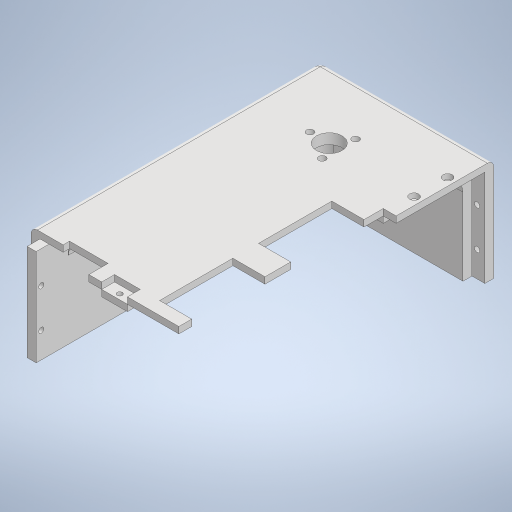
# Autodesk Inventor part: top_2
Saved by Autodesk Inventor 2023 (Build 270158000, 158)
## iProperties
Created: 2024-04-26
Part Number: top_2
Material: 常规
Document SubType Name: Modeling
Designer: Nitrene.P.L
Density: 1 g/cm^3
Appearance: 默认
Author: Nitrene.P.L
Autodesk Inventor part; units mm, degrees
ref_plane "YZ Plane" through (0, 0, 0) normal (1, 0, 0) x (0, 1, 0)
ref_plane "XZ Plane" through (0, 0, 0) normal (0, 1, 0) x (-1, 0, 0)
ref_plane "XY Plane" through (0, 0, 0) normal (0, 0, 1) x (1, 0, 0)
sketch "草图6" plane through (0, 0, 0) normal (0, 1, 0) x (-1, 0, 0)
  line L0 (125, 235) -> (-125, 235)
  line L1 (-125, 235) -> (-125, -235)
  line L2 (-125, -235) -> (125, -235)
  line L3 (125, -235) -> (125, 235)
  line L4 (0, 3) -> (0, -5)
  line L5 (3.5058, 0) -> (-3.4421, 0)
  line L6 (25, 144) -> (-32, 144)
  line L7 (-32, 144) -> (-32, 87)
  line L8 (-32, 87) -> (25, 87)
  line L9 (25, 87) -> (25, 144)
  line L10 (25, 67) -> (-32, 67)
  line L11 (-32, 67) -> (-32, 10)
  line L12 (-32, 10) -> (25, 10)
  line L13 (25, 10) -> (25, 67)
  line L14 (25, -10) -> (-32, -10)
  line L15 (-32, -10) -> (-32, -67)
  line L16 (-32, -67) -> (25, -67)
  line L17 (25, -67) -> (25, -10)
  line L18 (25, -87) -> (-32, -87)
  line L19 (-32, -87) -> (-32, -144)
  line L20 (-32, -144) -> (25, -144)
  line L21 (25, -144) -> (25, -87)
  line L22 (-66, 100) -> (-95, 100)
  line L23 (-95, 100) -> (-95, 54)
  line L24 (-95, 54) -> (-66, 54)
  line L25 (-66, 54) -> (-66, 100)
  line L26 (-66, -54) -> (-95, -54)
  line L27 (-95, -54) -> (-95, -100)
  line L28 (-95, -100) -> (-66, -100)
  line L29 (-66, -100) -> (-66, -54)
  line L30 (100, 15) -> (70, 15)
  line L31 (70, 15) -> (70, -15)
  line L32 (70, -15) -> (100, -15)
  line L33 (100, -15) -> (100, 15)
  circle A0 centre (65, 182) radius 10
  circle A1 centre (65, -182) radius 10
  circle A2 centre (65, 182) radius 15
  circle A3 centre (80, 182) radius 1.5
  circle A4 centre (57.5, 194.9904) radius 1.5
  circle A5 centre (57.5, 169.0096) radius 1.5
  line L34 (125, 235) -> (0, 235)
  line L35 (0, 235) -> (0, 0)
  line L36 (0, 0) -> (125, 0)
  line L37 (125, 0) -> (125, 235)
  line L38 (-125, 235) -> (0, 235)
  line L39 (0, 235) -> (0, 0)
  line L40 (0, 0) -> (-125, 0)
  line L41 (-125, 0) -> (-125, 235)
  line L42 (-125, -235) -> (0, -235)
  line L43 (0, -235) -> (0, 0)
  line L44 (0, 0) -> (-125, 0)
  line L45 (-125, 0) -> (-125, -235)
  line L46 (125, -235) -> (0, -235)
  line L47 (0, -235) -> (0, 0)
  line L48 (0, 0) -> (125, 0)
  line L49 (125, 0) -> (125, -235)
  circle A6 centre (65, -182) radius 15
  circle A7 centre (80, -182) radius 1.5
  circle A8 centre (57.5, -169.0096) radius 1.5
  circle A9 centre (57.5, -194.9904) radius 1.5
  point P0 (70, 0)
  point P1 (0, -10)
  point P2 (0, -67)
  point P3 (0, -87)
  point P4 (0, -144)
  point P5 (0, -235)
  point P6 (100, 0)
  dimension "d153" = 30
  dimension "d156" = 30
  dimension "d122" = 470
  dimension "d123" = 250
  dimension "d124" = 57
  dimension "d125" = 57
  dimension "d126" = 57
  dimension "d127" = 57
  dimension "d128" = 57
  dimension "d129" = 57
  dimension "d130" = 57
  dimension "d131" = 57
  dimension "d132" = 91
  dimension "d133" = 20
  dimension "d134" = 20
  dimension "d135" = 20
  dimension "d136" = 93
  dimension "d137" = 29
  dimension "d138" = 46
  dimension "d139" = 46
  dimension "d140" = 135
  dimension "d141" = 108
  dimension "d142" = 30
  dimension "d143" = 30
  dimension "d144" = 30
  dimension "d145" = 25
  dimension "d146" = 220
  dimension "d147" = 20
  dimension "d148" = 53
  dimension "d149" = 60
  dimension "d150" = 20
  dimension "d151" = 53
  dimension "d152" = 60
  dimension "d154" = 3
  dimension "d155" = 360
  dimension "d157" = 3
  dimension "d158" = 360
  constraints: 100 end point, 24 parallel, 14 horizontal, 12 perpendicular, 8 centre point, 3 collinear, 2 coincident, 2 horizontal alignment, 2 point on line, 2 vertical, 20 other
  measures "d122" distance of L3.start L3.end
  measures "d123" distance of L3.end L1.start
  measures "d124" distance of L8.end L8.start
  measures "d125" distance of L8.start L6.end
  measures "d126" distance of L13.start L11.end
  measures "d127" distance of L11.end L11.start
  measures "d128" distance of L16.end L15.end
  measures "d129" distance of L15.end L14.end
  measures "d130" distance of L20.end L19.end
  measures "d131" distance of L19.end L19.start
  measures "d132" distance between parallel lines of L0 L6
  measures "d133" distance between parallel lines of L10 L8
  measures "d134" distance between parallel lines of L12 L14
  measures "d135" distance between parallel lines of L18 L16
  measures "d136" distance between parallel lines of L1 L7
  measures "d137" distance of L25.start L23.end
  measures "d138" distance of L23.end L22.end
  measures "d139" distance of L27.end L27.start
  measures "d140" distance between parallel lines of L0 L22
  measures "d141" distance between parallel lines of L26 L24
  measures "d142" distance between parallel lines of L1 L23
  measures "d143" distance of L32.end L31.end
  measures "d144" distance of L31.end L31.start
  measures "d145" distance between parallel lines of L3 L33
  measures "d146" distance between parallel lines of L0 L30
  measures "d147" diameter of A0
  measures "d148" distance from line of L0 A0.centre
  measures "d149" distance from line of L3 A0.centre
  measures "d150" diameter of A1
  measures "d151" distance from line of L2 A1.centre
  measures "d152" distance from line of L3 A1.centre
  measures "d154" diameter of A3
  measures "d157" diameter of A7
extrude "拉伸5" add sketch "草图6" along normal blind 10 contours L3 L2 L43 L20 L21 L18 L16 L17 L14 L4 L5 L36 L31 L32 L33 | A7 A6 A9 A8
sketch "草图7" plane through (0, 0, 0) normal (0, -1, 0) x (1, 0, 0)
  line L0 (-70, 0) -> (0, 0) projected
  line L1 (0, 0) -> (-40, 0)
  line L2 (-40, 0) -> (-40, -159)
  line L3 (-40, -159) -> (0, -159)
  line L4 (0, -159) -> (0, 0)
  line L5 (-25, -144) -> (0, -144) projected
  line L6 (-25, -87) -> (-25, -144) projected
  line L7 (-60, 0) -> (-111, 0)
  line L8 (-111, 0) -> (-111, -25)
  line L9 (-111, -25) -> (-60, -25)
  line L10 (-60, -25) -> (-60, 0)
  line L11 (-70, -15) -> (-70, 0) projected
  line L12 (-100, -15) -> (-70, -15) projected
  line L13 (-100, 0) -> (-100, -15) projected
  dimension "d161" = 15
  dimension "d162" = 15
  dimension "d163" = 10
  dimension "d164" = 10
  dimension "d165" = 11
  constraints: 16 end point, 4 parallel, 2 horizontal, 2 perpendicular, 1 point on line
  measures "d161" distance between parallel lines of L5 L3
  measures "d162" distance between parallel lines of L6 L2
  measures "d163" distance between parallel lines of L10 L11
  measures "d164" distance between parallel lines of L9 L12
  measures "d165" distance between parallel lines of L13 L8
extrude "拉伸6" cut sketch "草图7" against normal blind 5 contours L0 L10 L9 L8 L7 L13 L12 L11 | L0 L4 L3 L2
sketch "草图8" plane through (0, 0, 0) normal (0, -1, 0) x (1, 0, 0)
  line L0 (-125, 0) -> (-111, 0) projected
  line L1 (-125, -235) -> (-125, 0) projected
  line L2 (-111, 0) -> (-125, 0)
  line L3 (-125, 0) -> (-125, -235)
  line L4 (-125, -235) -> (-111, -235)
  line L5 (-111, -235) -> (-111, 0)
  line L6 (0, -235) -> (-125, -235) projected
  line L7 (0, -235) -> (-125, -235)
  line L8 (-125, -235) -> (-125, -221)
  line L9 (-125, -221) -> (0, -221)
  line L10 (0, -221) -> (0, -235)
  point P0 (0, 0)
  point P1 (-111, -221)
  dimension "d168" = 14
  constraints: 16 end point, 4 parallel, 2 horizontal, 2 perpendicular, 1 point on line
  measures "d168" distance of L7.end L8.end
extrude "拉伸7" add sketch "草图8" along normal blind 70
sketch "草图11" plane through (0, 10, 0) normal (0, 1, 0) x (1, 0, 0)
  line L0 (-60, 0) -> (-60, 25) projected
  line L1 (-60, 0) -> (-40, 0)
  line L2 (-40, 0) -> (-40, 10)
  line L3 (-40, 10) -> (-60, 10)
  line L4 (-60, 10) -> (-60, 0)
  line L5 (-100, 0) -> (-100, 15) projected
  line L6 (-125, 235) -> (-125, 0) projected
  line L7 (-100, 0) -> (-125, 0)
  line L8 (-125, 0) -> (-125, 10)
  line L9 (-125, 10) -> (-100, 10)
  line L10 (-100, 10) -> (-100, 0)
  point P0 (0, 0)
  dimension "d178" = 10
  dimension "d179" = 20
  dimension "d187" = 10
  constraints: 16 end point, 4 parallel, 2 horizontal, 2 perpendicular, 1 point on line
  measures "d178" distance of L2.end L1.end
  measures "d179" distance between parallel lines of L0 L2
  measures "d187" distance of L7.end L8.end
extrude "拉伸9" cut sketch "草图11" against normal blind 5
sketch "草图12" plane through (0, 5, 0) normal (0, 1, 0) x (1, 0, 0)
  circle A0 centre (-50, 4) radius 2.1
  line L0 (-40, 0) -> (-60, 0) projected
  line L1 (-40, 10) -> (-40, 0) projected
  point P0 (0, 0)
  dimension "d182" = 4.2
  dimension "d183" = 4
  dimension "d184" = 10
  constraints: 1 centre point
  measures "d182" diameter of A0
  measures "d183" distance from line of L0 A0.centre
  measures "d184" distance from line of L1 A0.centre
extrude "拉伸10" cut sketch "草图12" against normal blind 5
sketch "草图13" plane through (-125, -70, -235) normal (-1, 0, 0) x (0, 0, 1)
  line L0 (235, 75) -> (225, 75) projected
  line L1 (235, 75) -> (225, 75)
  line L2 (225, 75) -> (225, 0)
  line L3 (225, 0) -> (235, 0)
  line L4 (235, 0) -> (235, 75)
  point P0 (235, 70)
  dimension "d188" = 10
  constraints: 8 end point, 2 parallel, 1 horizontal, 1 perpendicular
  measures "d188" distance between parallel lines of L2 L4
extrude "拉伸11" cut sketch "草图13" against normal blind 7
sketch "草图14" plane through (-118, -70, -235) normal (-1, 0, 0) x (0, 0, 1)
  circle A0 centre (231, 50) radius 2.1
  circle A1 centre (231, 20) radius 2.1
  line L0 (0, 80) -> (225, 80) projected
  line L1 (225, 0) -> (0, 0) projected
  line L2 (235, 75) -> (235, 0) projected
  point P0 (235, 70)
  dimension "d191" = 4.2
  dimension "d192" = 4.2
  dimension "d193" = 30
  dimension "d194" = 20
  dimension "d195" = 4
  dimension "d196" = 4
  constraints: 2 centre point
  measures "d191" diameter of A0
  measures "d192" diameter of A1
  measures "d193" distance from line of L0 A0.centre
  measures "d194" distance from line of L1 A1.centre
  measures "d195" distance from line of L2 A0.centre
  measures "d196" distance from line of L2 A1.centre
extrude "拉伸12" cut sketch "草图14" against normal blind 7
fillet "圆角1" radius 10 3 edges at (-111, 0, -123) (-111, -35, -221) (-55.5, 0, -221)
sketch "草图15" plane through (0, 10, 0) normal (0, 1, 0) x (1, 0, 0)
  line L0 (0, 159) -> (0, 211) projected
  line L1 (0, 159) -> (10, 159)
  line L2 (10, 159) -> (10, 235)
  line L3 (10, 235) -> (0, 235)
  line L4 (0, 235) -> (0, 159)
  circle A0 centre (4, 179) radius 2.1
  circle A1 centre (4, 205) radius 2.1
  point P0 (0, 0)
  point P1 (0, 211)
  dimension "d201" = 10
  dimension "d202" = 4.2
  dimension "d203" = 4.2
  dimension "d204" = 6
  dimension "d205" = 6
  dimension "d206" = 76
  dimension "d207" = 30
  dimension "d208" = 20
  constraints: 8 end point, 2 centre point, 2 parallel, 1 horizontal, 1 perpendicular
  measures "d201" distance of L3.end L2.end
  measures "d202" diameter of A0
  measures "d203" diameter of A1
  measures "d204" distance from line of L2 A0.centre
  measures "d205" distance from line of L2 A1.centre
  measures "d206" distance between parallel lines of L3 L1
  measures "d207" distance from line of L3 A1.centre
  measures "d208" distance from line of L1 A0.centre
extrude "拉伸13" add sketch "草图15" against normal blind 5
sketch "草图16" plane through (0, -70, -235) normal (0, 0, -1) x (-1, 0, 0)
  line L0 (-10, 75) -> (0, 75) projected
  line L1 (0, 60) -> (0, 0) projected
  line L2 (-10, 75) -> (0, 75)
  line L3 (0, 75) -> (0, 0)
  line L4 (0, 0) -> (-10, 0)
  line L5 (-10, 0) -> (-10, 75)
  circle A0 centre (-4, 50) radius 2.1
  circle A1 centre (-4, 20) radius 2.1
  line L6 (-10, 80) -> (125, 80) projected
  line L7 (125, 0) -> (0, 0) projected
  point P0 (0, 70)
  point P1 (0, 75)
  dimension "d211" = 4.2
  dimension "d212" = 4.2
  dimension "d213" = 30
  dimension "d214" = 20
  dimension "d215" = 6
  dimension "d216" = 6
  constraints: 8 end point, 2 centre point, 2 parallel, 1 horizontal, 1 perpendicular
  measures "d211" diameter of A0
  measures "d212" diameter of A1
  measures "d213" distance from line of L6 A0.centre
  measures "d214" distance from line of L7 A1.centre
  measures "d215" distance from line of L5 A0.centre
  measures "d216" distance from line of L5 A1.centre
extrude "拉伸14" add sketch "草图16" against normal blind 7
sketch "草图17" plane through (0, 10, 0) normal (0, 1, 0) x (1, 0, 0)
  circle A0 centre (4, 179) radius 2.1 projected
  circle A1 centre (4, 179) radius 3.6
  circle A2 centre (4, 205) radius 2.1 projected
  circle A3 centre (4, 205) radius 3.6
  point P0 (0, 0)
  dimension "d219" = 7.2
  dimension "d220" = 7.2
  constraints: 2 centre point, 2 coincident
  measures "d219" diameter of A1
  measures "d220" diameter of A3
extrude "拉伸15" cut sketch "草图17" against normal blind 4
sketch "草图18" plane through (-125, -70, -235) normal (0, 0, -1) x (-1, 0, 0)
  circle A0 centre (-129, 50) radius 2.1 projected
  circle A1 centre (-129, 50) radius 3.6
  circle A2 centre (-129, 20) radius 2.1 projected
  circle A3 centre (-129, 20) radius 3.6
  point P0 (-125, 70)
  dimension "d223" = 7.2
  dimension "d224" = 7.2
  constraints: 2 centre point, 2 coincident
  measures "d223" diameter of A1
  measures "d224" diameter of A3
extrude "拉伸16" cut sketch "草图18" against normal blind 4
fillet "圆角3" radius 5 3 edges at (-57.5, 10, -235) (-125, 10, -122.5) (-125, -30, -235)
sketch "草图19" plane through (0, 10, 0) normal (0, 1, 0) x (1, 0, 0)
  circle A0 centre (-80, 182) radius 1.5 projected
  circle A1 centre (-80, 182) radius 2.8
  circle A2 centre (-57.5, 194.9904) radius 1.5 projected
  circle A3 centre (-57.5, 194.9904) radius 2.8
  circle A4 centre (-57.5, 169.0096) radius 1.5 projected
  circle A5 centre (-57.5, 169.0096) radius 2.8
  point P0 (0, 0)
  dimension "d228" = 5.6
  dimension "d229" = 5.6
  dimension "d230" = 5.6
  constraints: 3 centre point, 3 coincident
  measures "d228" diameter of A1
  measures "d229" diameter of A3
  measures "d230" diameter of A5
extrude "拉伸17" cut sketch "草图19" against normal blind 3.1
sketch "草图20" plane through (0, 0, 0) normal (0, -1, 0) x (1, 0, 0)
  circle A0 centre (-65, -182) radius 10 projected
  circle A1 centre (-65, -182) radius 20
  point P0 (0, 0)
  dimension "d233" = 40
  constraints: 1 centre point, 1 coincident
  measures "d233" diameter of A1
extrude "拉伸18" cut sketch "草图20" against normal blind 5
sketch "草图21" plane through (-65, 5, -182) normal (0, -1, 0) x (1, 0, 0)
  circle A0 centre (0, 0) radius 20 projected
  circle A1 centre (0, 0) radius 20
  circle A2 centre (7.5, 12.9904) radius 1.5 projected
  circle A3 centre (7.5, 12.9904) radius 1.5
  circle A4 centre (7.5, -12.9904) radius 1.5 projected
  circle A5 centre (7.5, -12.9904) radius 1.5
  circle A6 centre (-15, 0) radius 1.5 projected
  circle A7 centre (-15, 0) radius 1.5
  circle A8 centre (0, 0) radius 10
  point P0 (65, 182)
  constraints: 5 centre point, 5 coincident
extrude "拉伸20" add sketch "草图21" along normal blind 3
sketch "草图22" plane through (-57.5, 6.9, -169.0096) normal (0, 1, 0) x (1, 0, 0)
  circle A0 centre (0, 0) radius 1.5 projected
  circle A1 centre (0, 0) radius 2.8
  circle A2 centre (-22.5, 12.9904) radius 2.8 projected
  circle A3 centre (-22.5, 12.9904) radius 2.8
  circle A4 centre (0, 25.9808) radius 2.8 projected
  circle A5 centre (0, 25.9808) radius 2.8
  point P0 (57.5, -169.0096)
  constraints: 3 centre point, 3 coincident
extrude "拉伸21" cut sketch "草图22" against normal blind 3 contours A0 | A1 | A2 | A4
